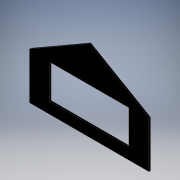
# Autodesk Inventor part: BA10
Saved by Autodesk Inventor 2017 (Build 210142000, 142)
## iProperties
Created: 2018-10-18
Part Number: BA10
Material: ABS Plastic
Document SubType Name: Modeling
Designer: Dell
Density: 1.06 g/cm^3
Appearance: Smooth - Black
Author: Dell
Autodesk Inventor part; units mm, degrees
ref_plane "YZ Plane" through (0, 0, 0) normal (1, 0, 0) x (0, 1, 0)
ref_plane "XZ Plane" through (0, 0, 0) normal (0, 1, 0) x (-1, 0, 0)
ref_plane "XY Plane" through (0, 0, 0) normal (0, 0, 1) x (1, 0, 0)
sketch "Sketch1" plane through (0, 0, 0) normal (0, 0, 1) x (1, 0, 0)
  line L0 (0, 0) -> (525.78, 0)
  line L1 (525.78, 0) -> (525.78, 205.6254)
  line L2 (525.78, 205.6254) -> (0, 205.6254)
  line L3 (0, 205.6254) -> (0, 0)
  line L4 (0, 205.6254) -> (262.89, 357.405)
  line L5 (262.89, 357.405) -> (525.78, 205.6254)
  point P0 (262.89, 205.6254)
  dimension "d0" = 525.78
  dimension "d1" = 205.6254
  dimension "d2" = 30
  constraints: 12 end point, 2 parallel, 1 horizontal, 1 midpoint, 1 perpendicular, 1 vertical alignment
  measures "d0" distance of L1.end L2.end
  measures "d1" distance of L0.end L1.end
  measures "d2" angle of L2 L5
extrude "Extrusion1" add sketch "Sketch1" along normal blind 6.35
sketch "Sketch5" plane through (0, 0, 6.35) normal (0, 0, 1) x (1, 0, 0)
  line L0 (87.89, 50) -> (437.89, 50)
  line L1 (437.89, 50) -> (437.89, 200)
  line L2 (437.89, 200) -> (87.89, 200)
  line L3 (87.89, 200) -> (87.89, 50)
  line L4 (0, 0) -> (525.78, 0) projected
  point P0 (262.89, 200)
  point P1 (262.89, 357.405)
  dimension "d16" = 350
  dimension "d17" = 150
  dimension "d21" = 50
  constraints: 8 end point, 2 parallel, 1 horizontal, 1 midpoint, 1 perpendicular, 1 vertical alignment
  measures "d16" distance of L1.end L2.end
  measures "d17" distance of L0.end L1.end
  measures "d21" distance between parallel lines of L4 L0
extrude "Extrusion5" cut sketch "Sketch5" against normal through all
body "Solid1"
